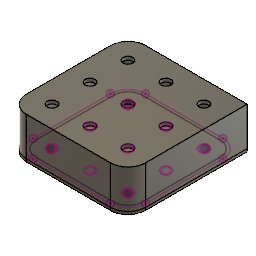
MidiControllerV3 (Autodesk Fusion 360 design; units mm, degrees)
Autodesk Fusion 360 part; units mm, degrees
sketch "Sketch1" plane through (0, 0, 0) normal (0, 1, 0) x (1, 0, 0)
  line L0 (0, 0) -> (80, 0)
  line L1 (80, 0) -> (80, -80)
  line L2 (80, -80) -> (0, -80)
  line L3 (0, -80) -> (0, 0)
  circle A0 centre (13, -13) radius 3.5
  circle A1 centre (40, -13) radius 3.5
  circle A2 centre (67, -13) radius 3.5
  circle A3 centre (13, -40) radius 3.5
  circle A4 centre (40, -40) radius 3.5
  circle A5 centre (67, -40) radius 3.5
  circle A6 centre (13, -67) radius 3.5
  circle A7 centre (40, -67) radius 3.5
  circle A8 centre (67, -67) radius 3.5
  line L4 (82.4, -82.4) -> (-2.4, -82.4)
  line L5 (-2.4, -82.4) -> (-2.4, 2.4)
  line L6 (-2.4, 2.4) -> (82.4, 2.4)
  line L7 (82.4, 2.4) -> (82.4, -82.4)
  dimension "d1" = 7
  dimension "d4" = 27
  dimension "d5" = -27
  dimension "d6" = 13
  dimension "d7" = 13
  dimension "d8" = 13
  dimension "d9" = 13
  dimension "d10" = -2.4
  constraint horizontal L0
  constraint vertical L1
  constraint horizontal L2
  constraint vertical L3
  constraint coincident L0.start L3.end
  measures "d1" diameter of A0
  measures "d6" distance of L0 A0.centre
  measures "d7" distance of L3 A0.centre
  measures "d8" distance of L1 A2.centre
  measures "d9" distance of L2 A8.centre
extrude "Extrude1" add sketch "Sketch1" along normal blind 2.4 contours L0 L1 L2 L3 | L4 L5 L6 L7 makes body 1
extrude "Extrude2" add sketch "Sketch1" against normal blind 25 contours L4 L5 L6 L7 bodies 1
fillet "Fillet1" radius 12.5 7 edges at (80, -12.5, 0) (-2.4, -11.3, 82.4) (-2.4, -11.3, -2.4) (82.4, -11.3, 82.4) (80, -12.5, 80) (0, -12.5, 80) (0, -12.5, 0) on bodies 1
sketch "Sketch2" plane through (0, -25, 0) normal (0, -1, 0) x (1, 0, 0)
  arc A0 (82.4, 69.9) -> (69.9, 82.4) centre (69.9, 69.9) ccw
  line L0 (69.9, 82.4) -> (10.1, 82.4)
  arc A1 (10.1, 82.4) -> (-2.4, 69.9) centre (10.1, 69.9) ccw
  line L1 (-2.4, 69.9) -> (-2.4, 10.1)
  arc A2 (-2.4, 10.1) -> (10.1, -2.4) centre (10.1, 10.1) ccw
  line L2 (10.1, -2.4) -> (82.4, -2.4)
  line L3 (82.4, -2.4) -> (82.4, 69.9)
  line L4 (12.5, 80) -> (67.5, 80)
  arc A3 (80, 67.5) -> (67.5, 80) centre (67.5, 67.5) ccw
  line L5 (80, 67.5) -> (80, 12.5)
  arc A4 (67.5, 0) -> (80, 12.5) centre (67.5, 12.5) ccw
  line L6 (67.5, 0) -> (12.5, 0)
  arc A5 (0, 12.5) -> (12.5, 0) centre (12.5, 12.5) ccw
  line L7 (0, 12.5) -> (0, 67.5)
  arc A6 (12.5, 80) -> (0, 67.5) centre (12.5, 67.5) ccw
  arc A7 (0, 12.5) -> (12.5, 0) centre (12.5, 12.5) ccw
  line L8 (12.5, 0) -> (67.5, 0)
  arc A8 (67.5, 0) -> (80, 12.5) centre (67.5, 12.5) ccw
  line L9 (80, 12.5) -> (80, 67.5)
  arc A9 (80, 67.5) -> (67.5, 80) centre (67.5, 67.5) ccw
  line L10 (67.5, 80) -> (12.5, 80)
  arc A10 (12.5, 80) -> (0, 67.5) centre (12.5, 67.5) ccw
  line L11 (0, 67.5) -> (0, 12.5)
  circle A11 centre (40, 67) radius 3.5
  circle A12 centre (67, 67) radius 3.5
  circle A13 centre (40, 40) radius 3.5
  circle A14 centre (67, 40) radius 3.5
  circle A15 centre (13, 67) radius 3.5
  circle A16 centre (13, 40) radius 3.5
  circle A17 centre (67, 13) radius 3.5
  circle A18 centre (40, 13) radius 3.5
  circle A19 centre (13, 13) radius 3.5
  line L12 (12.5, 2) -> (67.5, 2)
  arc A20 (67.5, 2) -> (78, 12.5) centre (67.5, 12.5) ccw
  line L13 (78, 12.5) -> (78, 67.5)
  arc A21 (78, 67.5) -> (67.5, 78) centre (67.5, 67.5) ccw
  line L14 (67.5, 78) -> (12.5, 78)
  arc A22 (12.5, 78) -> (2, 67.5) centre (12.5, 67.5) ccw
  line L15 (2, 67.5) -> (2, 12.5)
  arc A23 (2, 12.5) -> (12.5, 2) centre (12.5, 12.5) ccw
  dimension "d17" = -2
extrude "Extrude3" add sketch "Sketch2" along normal blind 2 separate body contours A0 L0 A1 L1 A2 L2 L3 | L4 A3 L5 A4 L6 A5 L7 A6 A7 L8 A8 L9 A9 L10 A10 L11 | A11 | A12 | A13 | A14 | A15 | A16 | A17 | A18 | A19 | L12 A20 L13 A21 L14 A22 L15 A23 makes body 2
extrude "Extrude4" add sketch "Sketch2" against normal blind 3 contours L4 A3 L5 A4 L6 A5 L7 A6 A7 L8 A8 L9 A9 L10 A10 L11 bodies 2
fillet "Fillet2" radius 3 8 edges at (2, -25, 40) (5.0754, -25, 74.9246) (40, -25, 78) (74.9246, -25, 74.9246) (78, -25, 40) (74.9246, -25, 5.0754) (40, -25, 2) (5.0754, -25, 5.0754) on bodies 2
chamfer "Chamfer1" distance 0.5 distance2 3 8 edges at (80, -22, 40) (76.3388, -22, 3.6612) (40, -22, 0) (3.6612, -22, 3.6612) (0, -22, 40) (3.6612, -22, 76.3388) (40, -22, 80) (76.3388, -22, 76.3388) measured on face at (30.8333, -22, 1.3333) measured on face at (30.8333, -22, 1.3333) measured on face at (30.8333, -22, 1.3333) measured on face at (30.8333, -22, 1.3333) measured on face at (30.8333, -22, 1.3333) measured on face at (30.8333, -22, 1.3333) measured on face at (30.8333, -22, 1.3333) measured on face at (30.8333, -22, 1.3333) on bodies 2
sketch "Sketch3" plane through (-2.4, 0, 0) normal (-1, 0, 0) x (0, 0, 1)
  line L0 (10.1, 2.4) -> (10.1, -25)
  line L1 (10.1, -25) -> (69.9, -25)
  line L2 (69.9, -25) -> (69.9, 2.4)
  line L3 (69.9, 2.4) -> (10.1, 2.4)
  line L4 (45, -24) -> (35, -24)
  line L5 (35, -24) -> (35, -16)
  line L6 (35, -16) -> (45, -16)
  line L7 (45, -16) -> (45, -24)
  line L8 (45, -24) -> (35, -16) construction
  line L9 (35, -24) -> (45, -16) construction
  line L10 (40, -25) -> (40, -20) construction
  point P0 (40, -20)
  point P1 (40, -25)
  dimension "d25" = 10
  dimension "d26" = 8
  dimension "d27" = 5
  constraint perpendicular L4 L5
  constraint parallel L4 L6
  constraint parallel L5 L7
  constraint horizontal L4
  constraint coincident L8 P0
  constraint coincident L9 P0
  constraint coincident P1 L10.start
  constraint coincident P0 L10.end
  constraint vertical L10
  measures "d25" distance of L5.end L6.end
  measures "d26" distance of L4.end L5.end
  measures "d27" distance of P1 P0
extrude "Extrude5" cut sketch "Sketch3" against normal blind 12 contours L4 L5 L6 L7 bodies 1 2
chamfer "Chamfer2" distance 8 distance2 2 2 edges at (1.25, -22, 45) (1.25, -22, 35) measured on face at (79.0001, -22, 30.8333) measured on face at (79.0001, -22, 30.8333) on bodies 2
extrude "Extrude8" cut 1 faces at (-1.6, -24, 38.3333) along direction (0, -1, 0) blind 9 on bodies 1 bodies 1
sketch "Sketch4" plane through (0, -27, 0) normal (0, -1, 0) x (1, 0, 0)
  line L0 (82.4, -2.4) -> (82.4, 69.9)
  arc A0 (82.4, 69.9) -> (69.9, 82.4) centre (69.9, 69.9) ccw
  line L1 (69.9, 82.4) -> (10.1, 82.4)
  arc A1 (10.1, 82.4) -> (-2.4, 69.9) centre (10.1, 69.9) ccw
  line L2 (-2.4, 69.9) -> (-2.4, 10.1)
  arc A2 (-2.4, 10.1) -> (10.1, -2.4) centre (10.1, 10.1) ccw
  line L3 (10.1, -2.4) -> (82.4, -2.4)
  circle A3 centre (72.8033, 72.8033) radius 25
  arc A4 (75, 67.5) -> (67.5, 75) centre (67.5, 67.5) ccw
  circle A5 centre (82.4, -2.4) radius 22.5
  circle A6 centre (5.0754, 74.9246) radius 25
  arc A7 (12.5, 78) -> (2, 67.5) centre (12.5, 67.5) ccw
  circle A8 centre (7.1967, 7.1967) radius 25
  arc A9 (5, 12.5) -> (12.5, 5) centre (12.5, 12.5) ccw
  dimension "d32" = 50
  dimension "d33" = 45
  dimension "d34" = 50
  dimension "d35" = 50
  constraint midpoint A3.centre A4
  constraint coincident L0.start L3.end
  constraint midpoint A6.centre A7
  constraint midpoint A8.centre A9
  measures "d32" diameter of A3
  measures "d33" diameter of A5
  measures "d34" diameter of A6
  measures "d35" diameter of A8
extrude "Extrude6" [suppressed]
sketch "Sketch5" plane through (0, 2.4, 0) normal (0, 1, 0) x (-1, 0, 0)
  arc A0 (-69.9, 82.4) -> (-82.4, 69.9) centre (-69.9, 69.9) ccw
  line L0 (-82.4, 69.9) -> (-82.4, -2.4)
  line L1 (-82.4, -2.4) -> (-10.1, -2.4)
  arc A1 (-10.1, -2.4) -> (2.4, 10.1) centre (-10.1, 10.1) ccw
  line L2 (2.4, 10.1) -> (2.4, 69.9)
  arc A2 (2.4, 69.9) -> (-10.1, 82.4) centre (-10.1, 69.9) ccw
  line L3 (-10.1, 82.4) -> (-69.9, 82.4)
  circle A3 centre (-40, 67) radius 3.5
  circle A4 centre (-67, 67) radius 3.5
  circle A5 centre (-40, 40) radius 3.5
  circle A6 centre (-67, 40) radius 3.5
  circle A7 centre (-13, 67) radius 3.5
  circle A8 centre (-13, 40) radius 3.5
  circle A9 centre (-67, 13) radius 3.5
  circle A10 centre (-40, 13) radius 3.5
  circle A11 centre (-13, 13) radius 3.5
  circle A12 centre (-82.4, -2.4) radius 25
  circle A13 centre (-78.7388, 78.7388) radius 25
  circle A14 centre (-1.2612, 78.7388) radius 25
  circle A15 centre (-1.2612, 1.2612) radius 25
  dimension "d38" = 50
  dimension "d39" = 50
  dimension "d40" = 50
  dimension "d41" = 50
  constraint coincident L0.end L1.start
  constraint midpoint A0 A13.centre
  constraint midpoint A2 A14.centre
  constraint midpoint A1 A15.centre
  measures "d38" diameter of A12
  measures "d39" diameter of A13
  measures "d40" diameter of A14
  measures "d41" diameter of A15
extrude "Extrude7" [suppressed]
equation "d6 = spacingoutside"
equation "d7 = spacingoutside"
equation "d8 = spacingoutside"
equation "d9 = spacingoutside"
equation "spacingoutside = 13 mm"
named bodies: "Box", "Lid"
